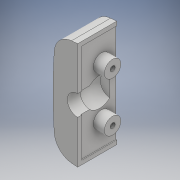
# Autodesk Inventor part: Part2
Saved by Autodesk Inventor 2017 (Build 210142000, 142)
## iProperties
Created: 2019-06-26
Part Number: Part2
Material: Generic
Document SubType Name: Modeling
Designer: Ole Simmering
Density: 1 g/cm^3
Appearance: Default
Author: Ole Simmering
Autodesk Inventor part; units mm, degrees
ref_plane "YZ Plane" through (0, 0, 0) normal (1, 0, 0) x (0, 1, 0)
ref_plane "XZ Plane" through (0, 0, 0) normal (0, 1, 0) x (-1, 0, 0)
ref_plane "XY Plane" through (0, 0, 0) normal (0, 0, 1) x (1, 0, 0)
sketch "Sketch1" plane through (0, 0, 0) normal (0, 1, 0) x (-1, 0, 0)
  line L0 (0, 0) -> (0, -26)
  line L1 (0, -26) -> (1.5, -25.8688)
  line L2 (-5, -13) -> (15, -13) construction
  line L3 (0, 0) -> (1.5, -0.1312)
  arc A0 (1.5, -25.8688) -> (5.6905, -21.6131) centre (1.0988, -21.2827) ccw
  arc A1 (5.6905, -4.3869) -> (1.5, -0.1312) centre (1.0988, -4.7173) ccw
  arc A2 (5.6905, -21.6131) -> (6, -13) centre (-114, -13) ccw
  arc A3 (6, -13) -> (5.6905, -4.3869) centre (-114, -13) ccw
  dimension "d0" = 26
  dimension "d1" = 85
  dimension "d2" = 1.5
  dimension "d3" = 6
  dimension "d4" = 120
  constraints: 8 end point, 8 point on circle, 4 centre point, 4 symmetric about line, 2 tangent, 1 coincident, 1 horizontal, 1 point on line, 1 vertical, 1 other
  measures "d0" distance of L0.start L0.end
  measures "d1" angle of L1 L0
  measures "d2" distance from line of L1.end L0
  measures "d3" distance from line of A2.end L0
  measures "d4" radius of A2
extrude "Extrusion1" add sketch "Sketch1" along normal blind 9.5
sketch "Sketch2" plane through (0, 0, 0) normal (1, 0, 0) x (0, 0, -1)
  circle A0 centre (7, 6) radius 2
  circle A1 centre (19, 6) radius 2
  line L0 (0, 0) -> (26, 0) construction
  line L1 (26, 0) -> (26, 9.5) construction
  line L2 (0, 9.5) -> (1, 9.5) construction
  line L3 (0, 0) -> (0, 9.5) construction
  line L4 (1, 9.5) -> (1, 1)
  line L5 (1, 1) -> (25, 1)
  line L6 (25, 1) -> (25, 9.5)
  line L7 (0, 0) -> (0, 9.5) construction
  line L8 (0, 9.5) -> (1, 9.5) construction
  line L9 (26, 0) -> (26, 9.5) construction
  line L10 (1, 9.5) -> (25, 9.5)
  line L11 (25, 9.5) -> (26, 9.5) construction
  dimension "d7" = 1
  dimension "d8" = 1
  dimension "d9" = 1
  constraints: 24 end point, 4 perpendicular, 2 centre point, 1 parallel, 1 point on line, 1 vertical
  measures "d7" distance between parallel lines of L3 L4
  measures "d8" distance between parallel lines of L0 L5
  measures "d9" distance between parallel lines of L1 L6
extrude "Extrusion2" cut sketch "Sketch2" against normal blind 0.2
sketch "Sketch3" plane through (0, 6, -7) normal (1, 0, 0) x (0, 0, -1)
  circle A0 centre (0, 0) radius 2 projected
  circle A1 centre (0, 0) radius 2
  circle A2 centre (12, 0) radius 2
  point P0 (-7, -6)
  constraints: 2 centre point, 1 coincident
extrude "Extrusion3" add sketch "Sketch3" along normal blind 2.5
sketch "Sketch4" plane through (2.5, 6, -7) normal (1, 0, 0) x (0, 0, -1)
  circle A0 centre (12, 0) radius 2 projected
  point P0 (-7, -6)
  point P1 (0, 0)
  constraints: 1 coincident
hole "Hole1" at (2.5, 6, -7) at (2.5, 6, -19) direction (-1, 0, 0) diameter 1.221 depth 5.3 tip angle 118 thread size "M1.6x0.35" class "6H" standard "ANSI Metric M Profile"
sketch "Sketch5" plane through (0, 0, 0) normal (1, 0, 0) x (0, 0, -1)
  line L0 (21.6131, 9.5) -> (4.3869, 9.5) construction
  line L1 (13, 9.5) -> (13, -3) construction
  line L2 (10.5, 8) -> (13, 8) construction
  arc A0 (15.5, 3.101) -> (15.5, 8) centre (13, 5.5505) ccw
  line L3 (21.6131, 0) -> (4.3869, 0) construction
  line L4 (10.5, 0) -> (10.5, 3.101) construction
  line L5 (15.5, 0) -> (15.5, 3.101)
  line L6 (13, 9.0505) -> (13, 8) construction
  arc A1 (13, 2.0505) -> (15.5, 3.101) centre (13, 5.5505) ccw construction
  arc A2 (13, 9.0505) -> (13, 2.0505) centre (13, 5.5505) ccw construction
  arc A3 (15.5, 8) -> (13, 9.0505) centre (13, 5.5505) ccw construction
  line L7 (13, 8) -> (15.5, 8)
  line L8 (13, 8) -> (13, 0)
  line L9 (13, 0) -> (15.5, 0)
  point P0 (0, 0)
  dimension "d24" = 1.5
  dimension "d25" = 5
  dimension "d26" = 7
  dimension "d27" = 5
  constraints: 16 end point, 12 point on circle, 6 point on line, 4 centre point, 3 horizontal, 2 midpoint, 1 parallel, 1 perpendicular, 1 symmetric about line, 1 vertical, 1 other
  measures "d24" distance between parallel lines of L0 L2
  measures "d25" distance of L2.start L7.end
  measures "d26" diameter of A0
  measures "d27" distance between parallel lines of L5 L4
revolve "Revolution1" cut sketch "Sketch5" angle 360 about axis through (0, 8, -13) along (0, -1, 0)
equation "\"d9\" = d7"
body "Solid1"
